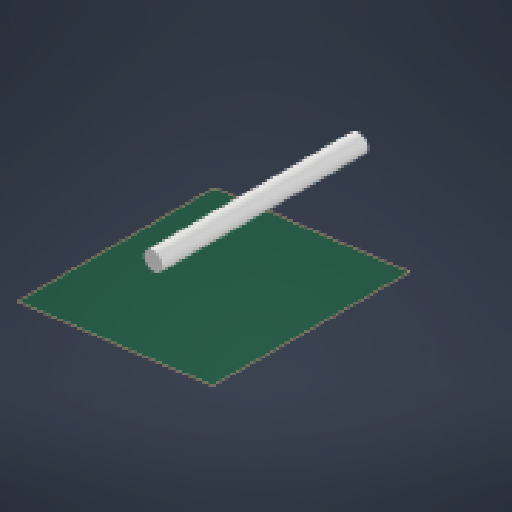
# Autodesk Inventor part: counter_shaft
Saved by Autodesk Inventor 2024 (Build 280153000, 153)
## iProperties
Created: 2026-03-30
Part Number: counter_shaft
Material: Generic
Document SubType Name: Modeling
Designer: schar
Density: 1 g/cm^3
Appearance: Default
Author: schar
Autodesk Inventor part; units mm, degrees
ref_plane "YZ Plane" through (0, 0, 0) normal (1, 0, 0) x (0, 1, 0)
ref_plane "XZ Plane" through (0, 0, 0) normal (0, 1, 0) x (-1, 0, 0)
ref_plane "XY Plane" through (0, 0, 0) normal (0, 0, 1) x (1, 0, 0)
sketch "Sketch1" plane through (0, 0, 0) normal (0, 0, 1) x (1, 0, 0)
  circle A0 centre (0, 0) radius 2.4837
  constraints: 1 centre point, 1 coincident
extrude "Extrusion1" add sketch "Sketch1" against normal blind 55
ref_plane "Work Plane1" through (11.0441, -3.6439, -6) normal (0.1253942, -0.992107, 0) x (-0.992107, -0.1253942, 0)
sketch "Sketch2" plane through (11.0441, -3.6439, -6) normal (0.1253942, -0.992107, 0) x (-0.992107, -0.1253942, 0)
  line L0 (12.9837, 49) -> (8.0163, 49) projected
  line L1 (10.5, 49) -> (10.5, 45)
  line L2 (10.5, 45) -> (10.5, 42)
  line L3 (8.5, 45) -> (12.5, 45)
  line L4 (12.5, 45) -> (12.5, 42)
  line L5 (12.5, 42) -> (8.5, 42)
  line L6 (8.5, 42) -> (8.5, 45)
  line L7 (8.5, 45) -> (12.5, 42) construction
  line L8 (12.5, 45) -> (8.5, 42) construction
  point P0 (10.5, -6)
  point P1 (10.5, 43.5)
  dimension "d2" = 4
  dimension "d3" = 3
  dimension "d4" = 4
  constraints: 16 end point, 4 midpoint, 2 parallel, 1 horizontal, 1 perpendicular, 1 point on line, 1 vertical
  measures "d2" distance of L1.start L1.end
  measures "d3" distance of L1.end L2.end
  measures "d4" distance of L4.end L5.end
extrude "Extrusion2" cut sketch "Sketch2" against normal blind 3.5
body "Solid1"
